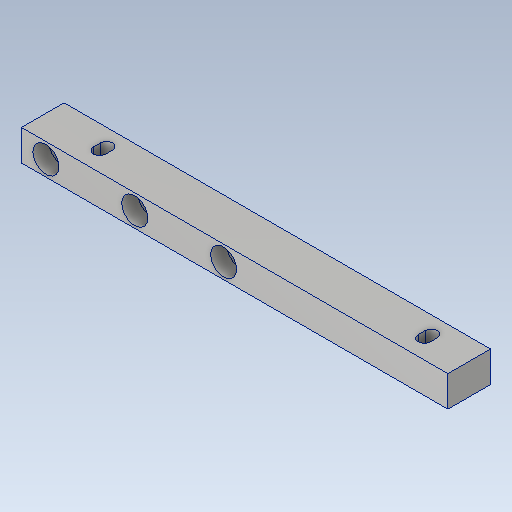
# Autodesk Inventor part: FAB-CAM001 - Filter Wheel Bracket
Saved by Autodesk Inventor 2020 (Build 240168000, 168)
## iProperties
Created: 2013-04-24
Part Number: FAB-CAM001 - Filter Wheel Bracket
Material: Aluminum 6061
Document SubType Name: Modeling
Designer: map
Density: 2.7 g/cm^3
Appearance: Aluminum - Flat
Mass: 101.063 g
Surface Area: 133.96 cm^2
Volume: 37.4306 cm^3
Sending System: SolidWorks 2015
Last Author: ml2377
Last Saved: 2016-03-24
Author: map
Autodesk Inventor part; units mm, degrees
ref_plane "YZ Plane" through (0, 0, 0) normal (1, 0, 0) x (0, 1, 0)
ref_plane "XZ Plane" through (0, 0, 0) normal (0, 1, 0) x (-1, 0, 0)
ref_plane "XY Plane" through (0, 0, 0) normal (0, 0, 1) x (1, 0, 0)
derived "__05_Detection_MASTER__.ipt"
sketch "Sketch1" plane through (0, 0, 0) normal (0, 0, 1) x (1, 0, 0)
  line L0 (-119.8204, -325) -> (119.8204, -325)
  line L1 (0, 0) -> (0, -325) construction
  line L2 (-50, -75) -> (50, -75)
  line L3 (50, -75) -> (50, -195)
  line L4 (50, -195) -> (-50, -195)
  line L5 (-50, -195) -> (-50, -75)
  line L6 (-22.9, -88) -> (114.26, -88)
  line L7 (-37.5, -94.5) -> (37.5, -94.5)
  line L8 (-40.82, -88) -> (132.18, -88) construction
  point P0 (0, -75)
  point P1 (0, -94.5)
  point P2 (0, -94.5)
  point P3 (45.68, -88)
sketch "Sketch7" plane through (0, 0, 0) normal (0, 0, 1) x (1, 0, 0)
  line L0 (-40.82, -88) -> (132.18, -88) construction
  line L1 (-40.82, -88) -> (132.18, -88)
  line L2 (132.18, -88) -> (132.18, -101)
  line L3 (132.18, -101) -> (-40.82, -101)
  line L4 (-40.82, -101) -> (-40.82, -88)
  line L5 (-40.82, -101) -> (-47.82, -101)
  line L6 (-47.82, -101) -> (-47.82, -88)
  line L7 (-47.82, -88) -> (-40.82, -88)
  line L8 (-40.82, -88) -> (-40.82, -101)
  line L9 (-37.5, -94.5) -> (37.5, -94.5) projected
  point P0 (0, 0)
  dimension "d49" = 7
  constraints: 16 end point, 4 parallel, 2 horizontal, 2 perpendicular, 1 collinear, 1 other
  measures "d49" distance of L7.end L6.end
extrude "Extrusion2" add sketch "Sketch7" against normal blind 18
hole "Hole7" at (0, 0, 0) at (-37.5, -94.5, 0) at (0, -94.5, 0) at (37.5, -94.5, 0) direction (0, 0, -1) diameter 6.6 end through all counterbore diameter 11 counterbore depth 6.8 clearance for "Socket Head Cap Screw ISO 4762" size "M6" standard "ISO"
sketch "Sketch8" plane through (-47.82, -101, 0) normal (0, -1, 0) x (1, 0, 0)
  line L0 (180, 0) -> (0, 0) construction
  line L1 (24.92, 0) -> (24.92, -18) construction
  line L2 (180, -18) -> (0, -18) construction
  line L3 (162.08, 0) -> (162.08, -14) construction
  line L4 (24.92, -8) -> (24.92, -11) construction
  line L5 (20.12, -8) -> (20.12, -11)
  line L6 (29.72, -11) -> (29.72, -8)
  arc A0 (29.72, -8) -> (20.12, -8) centre (24.92, -8) ccw
  arc A1 (20.12, -11) -> (29.72, -11) centre (24.92, -11) ccw
  line L7 (162.08, -8) -> (162.08, -11) construction
  line L8 (157.28, -8) -> (157.28, -11)
  line L9 (166.88, -11) -> (166.88, -8)
  arc A2 (166.88, -8) -> (157.28, -8) centre (162.08, -8) ccw
  arc A3 (157.28, -11) -> (166.88, -11) centre (162.08, -11) ccw
  line L10 (0, 0) -> (0, -18) construction
  line L11 (180, 0) -> (180, -18) construction
  line L12 (24.92, -9.5) -> (162.08, -9.5) construction
  point P0 (47.82, 0)
  dimension "d59" = 3
  dimension "d60" = 9.6
  dimension "d61" = 9.6
  dimension "d62" = 3
  dimension "d72" = 8.5
  constraints: 22 end point, 8 point on circle, 8 tangent, 5 point on line, 4 centre point, 2 midpoint, 2 parallel, 2 vertical, 1 horizontal
  measures "d59" distance of L4.start L4.end
  measures "d60" diameter of A1
  measures "d61" diameter of A3
  measures "d62" distance of L7.end L7.start
  measures "d72" distance between parallel lines of L12 L2
extrude "Extrusion3" cut sketch "Sketch8" against normal blind 5
sketch "Sketch9" plane through (-47.82, -96, 0) normal (0, -1, 0) x (1, 0, 0)
  line L0 (20.12, -11) -> (20.12, -8) projected
  arc A0 (20.12, -11) -> (29.72, -11) centre (24.92, -11) ccw projected
  line L1 (29.72, -8) -> (29.72, -11) projected
  arc A1 (29.72, -8) -> (20.12, -8) centre (24.92, -8) ccw projected
  line L2 (157.28, -11) -> (157.28, -8) projected
  arc A2 (157.28, -11) -> (166.88, -11) centre (162.08, -11) ccw projected
  line L3 (166.88, -8) -> (166.88, -11) projected
  arc A3 (166.88, -8) -> (157.28, -8) centre (162.08, -8) ccw projected
  line L4 (24.92, -8) -> (24.92, -11) construction
  line L5 (22.32, -8) -> (22.32, -11)
  line L6 (27.52, -11) -> (27.52, -8)
  arc A4 (27.52, -8) -> (22.32, -8) centre (24.92, -8) ccw
  arc A5 (22.32, -11) -> (27.52, -11) centre (24.92, -11) ccw
  line L7 (162.08, -8) -> (162.08, -11) construction
  line L8 (164.68, -8) -> (164.68, -11)
  line L9 (159.48, -11) -> (159.48, -8)
  arc A6 (164.68, -8) -> (159.48, -8) centre (162.08, -8) ccw
  arc A7 (159.48, -11) -> (164.68, -11) centre (162.08, -11) ccw
  point P0 (47.82, 0)
  point P1 (24.92, -9.5)
  point P2 (162.08, -9.5)
  dimension "d67" = 2.6
  dimension "d68" = 2.6
  constraints: 16 end point, 8 point on circle, 8 tangent, 4 centre point, 3 parallel, 2 midpoint, 1 vertical
  measures "d67" radius of A5
  measures "d68" radius of A7
extrude "Extrusion4" cut sketch "Sketch9" against normal through all contours A4 L6 A5 L5 | L8 A7 L9 A6
equation "\"d61\" = d60"
equation "\"d62\" = d59"
equation "\"d68\" = d67"
body "Solid4"
